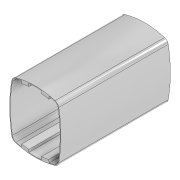
# Autodesk Inventor part: lineaire as deel 3
Saved by Autodesk Inventor 2020.3 (Build 243373000, 373)
## iProperties
Created: 2020-09-16
Part Number: lineaire as deel 3
Material: Aluminum 6061
Document SubType Name: Modeling
Designer: Svend
Density: 2.7 g/cm^3
Appearance: Aluminum - Polished
Author: Svend
Autodesk Inventor part; units mm, degrees
ref_plane "YZ Plane" through (0, 0, 0) normal (1, 0, 0) x (0, 1, 0)
ref_plane "XZ Plane" through (0, 0, 0) normal (0, 1, 0) x (-1, 0, 0)
ref_plane "XY Plane" through (0, 0, 0) normal (0, 0, 1) x (1, 0, 0)
sketch "Sketch1" plane through (0, 0, 0) normal (0, 0, 1) x (1, 0, 0)
  line L0 (-57, -57.5) -> (57, 57.5) construction
  line L1 (-67.5, 67.5) -> (67.5, 67.5) construction
  line L2 (67.5, 67.5) -> (67.5, -67.5) construction
  line L3 (67.5, -67.5) -> (-67.5, -67.5) construction
  line L4 (-67.5, -67.5) -> (-67.5, 67.5) construction
  line L5 (-67.5, 67.5) -> (67.5, -67.5) construction
  line L6 (67.5, 67.5) -> (-67.5, -67.5) construction
  circle A0 centre (-37.5, 37.5) radius 4
  circle A1 centre (-37.5, -37.5) radius 4
  circle A2 centre (37.5, -37.5) radius 4
  circle A3 centre (37.5, 37.5) radius 4
  arc A4 (-48.5, 62.5) -> (-48.5, -62.5) centre (326.325, 0) ccw
  line L7 (0, 67.5) -> (0, -67.5) construction
  line L8 (67.5, -67.5) -> (67.5, 67.5) construction
  arc A5 (48.5, -62.5) -> (48.5, 62.5) centre (-326.325, 0) ccw
  arc A6 (48.5, 62.5) -> (-48.5, 62.5) centre (0, -110.8429) ccw
  line L9 (-67.5, 0) -> (53.675, 0) construction
  arc A7 (-48.5, -62.5) -> (48.5, -62.5) centre (0, 110.8429) ccw
  arc A8 (-30.7003, 46.1842) -> (-30.7003, -46.1842) centre (326.325, 0) ccw
  arc A9 (-30.7003, -46.1842) -> (30.7003, -46.1842) centre (0, 110.8429) ccw
  arc A10 (30.7003, -46.1842) -> (30.7003, 46.1842) centre (-326.325, 0) ccw
  arc A11 (30.7003, 46.1842) -> (-30.7003, 46.1842) centre (0, -110.8429) ccw
  arc A12 (-55.5322, 68.7683) -> (-55.5322, -68.7683) centre (326.325, 0) ccw
  arc A13 (-55.5322, -68.7683) -> (55.5322, -68.7683) centre (0, 110.8429) ccw
  arc A14 (55.5322, -68.7683) -> (55.5322, 68.7683) centre (-326.325, 0) ccw
  arc A15 (55.5322, 68.7683) -> (-55.5322, 68.7683) centre (0, -110.8429) ccw
  arc A16 (-57.2838, 70.3161) -> (-57.2838, -70.3161) centre (326.325, 0) ccw
  arc A17 (-57.2838, -70.3161) -> (57.2838, -70.3161) centre (0, 110.8429) ccw
  arc A18 (57.2838, -70.3161) -> (57.2838, 70.3161) centre (-326.325, 0) ccw
  arc A19 (57.2838, 70.3161) -> (-57.2838, 70.3161) centre (0, -110.8429) ccw
  line L10 (18.657, 86.2762) -> (17.0881, 68.3442)
  line L11 (40.2153, 83.0301) -> (37.0881, 65.2948)
  line L12 (-18.657, 86.2762) -> (-17.0881, 68.3442)
  line L13 (-40.2153, 83.0301) -> (-37.0881, 65.2948)
  line L14 (18.657, -86.2762) -> (17.0881, -68.3442)
  line L15 (40.2153, -83.0301) -> (37.0881, -65.2948)
  line L16 (-40.2153, -83.0301) -> (-37.0881, -65.2948)
  line L17 (-18.657, -86.2762) -> (-17.0881, -68.3442)
  arc A20 (-64.266, 76.4373) -> (-64.266, -76.4373) centre (326.325, 0) ccw
  arc A21 (-64.266, -76.4373) -> (64.266, -76.4373) centre (0, 110.8429) ccw
  arc A22 (64.266, -76.4373) -> (64.266, 76.4373) centre (-326.325, 0) ccw
  arc A23 (64.266, 76.4373) -> (-64.266, 76.4373) centre (0, -110.8429) ccw
  arc A24 (-66.006, 77.9512) -> (-66.006, -77.9512) centre (326.325, 0) ccw
  arc A25 (-66.006, -77.9512) -> (66.006, -77.9512) centre (0, 110.8429) ccw
  arc A26 (66.006, -77.9512) -> (66.006, 77.9512) centre (-326.325, 0) ccw
  arc A27 (66.006, 77.9512) -> (-66.006, 77.9512) centre (0, -110.8429) ccw
  point P0 (0, 0)
  point P1 (0, 0)
  point P2 (-53.675, 0)
  point P3 (0, 0)
  point P4 (-17.7854, 76.314)
  point P5 (-38.478, 73.1774)
  point P6 (17.7854, -76.314)
  point P7 (38.478, -73.1774)
  point P8 (-38.478, -73.1774)
  point P9 (-17.7854, -76.314)
  point P10 (-38.478, 73.1774)
  point P11 (-17.7854, 76.314)
  point P12 (38.478, -73.1774)
  point P13 (17.7854, -76.314)
  point P14 (-17.7854, -76.314)
  point P15 (-38.478, -73.1774)
  point P16 (-17.9597, -78.3064)
  point P17 (-38.8255, -75.1479)
  point P18 (-38.8255, 75.1479)
  point P19 (-17.9597, 78.3064)
  point P20 (17.9597, 78.3064)
  point P21 (38.8255, 75.1479)
  point P22 (38.8255, -75.1479)
  point P23 (17.9597, -78.3064)
  dimension "d3" = 135
  dimension "d4" = 135
  dimension "d5" = 8
  dimension "d9" = 360
  dimension "d29" = 75
  dimension "d30" = 125
  dimension "d31" = 97
  dimension "d32" = 180
  dimension "d33" = 380
  dimension "d34" = 20
  dimension "d36" = 8
  dimension "d37" = 2
  dimension "d38" = 5
  dimension "d39" = 20
  dimension "d41" = 5
  dimension "d42" = 8
  dimension "d43" = 2
  constraints: 59 point on circle, 36 end point, 28 centre point, 13 symmetric about line, 7 midpoint, 7 point on line, 2 horizontal, 2 parallel, 1 coincident, 1 horizontal alignment, 1 perpendicular, 26 other
  measures "d3" distance of L2.end L3.end
  measures "d4" distance of L1.end L2.end
  measures "d5" diameter of A0
  measures "d29" distance of A0.centre A3.centre
  measures "d30" distance of A4.end A4.start
  measures "d31" distance of A5.end A4.start
  measures "d32" radius of A6
  measures "d33" radius of A4
  measures "d34" radial gap between concentric circles of A6 A11
  measures "d36" radial gap between concentric circles of A6 A15
  measures "d37" radial gap between concentric circles of A15 A19
  measures "d38" angle of L10 L11
  measures "d39" horizontal distance of L10.end L11.end
  measures "d41" angle of L7 L10
  measures "d42" radial gap between concentric circles of A19 A23
  measures "d43" radial gap between concentric circles of A23 A27
extrude "Extrusion1" add sketch "Sketch1" along normal mid plane 310 contours L13 A23 L12 A19 | A17 L17 A21 L16 | L10 A23 L11 A19 | A17 L15 A21 L14 | A27 A26 A25 A24
fillet "Fillet2" radius 15 8 edges at (64.266, 76.4373, 0) (-64.266, 76.4373, 0) (-64.266, -76.4373, 0) (64.266, -76.4373, 0) (-66.006, 77.9512, 0) (-66.006, -77.9512, 0) (66.006, -77.9512, 0) (66.006, 77.9512, 0)
sketch "Sketch4" plane through (0, 0, -155) normal (0, 0, -1) x (-1, 0, 0)
  arc A0 (67.6752, -69.0208) -> (67.6752, 69.0208) centre (-326.325, 0) ccw projected
  arc A1 (-57.1894, 80.8062) -> (-67.6752, 69.0208) centre (-52.9002, 66.4325) ccw projected
  arc A2 (-67.6752, 69.0208) -> (-67.6752, -69.0208) centre (326.325, 0) ccw projected
  arc A3 (-67.6752, -69.0208) -> (-57.1894, -80.8062) centre (-52.9002, -66.4325) ccw projected
  arc A4 (-57.1894, -80.8062) -> (57.1894, -80.8062) centre (0, 110.8429) ccw projected
  arc A5 (57.1894, -80.8062) -> (67.6752, -69.0208) centre (52.9002, -66.4325) ccw projected
  arc A6 (67.6752, -69.0208) -> (67.6752, 69.0208) centre (-326.325, 0) ccw projected
  arc A7 (67.6752, 69.0208) -> (57.1894, 80.8062) centre (52.9002, 66.4325) ccw projected
  arc A8 (57.1894, 80.8062) -> (-57.1894, 80.8062) centre (0, -110.8429) ccw projected
  line L0 (17.9597, -78.3064) -> (18.657, -86.2762) projected
  arc A9 (-18.657, -86.2762) -> (18.657, -86.2762) centre (0, 110.8429) ccw projected
  line L1 (-18.657, -86.2762) -> (-17.9597, -78.3064) projected
  arc A10 (-38.8255, -75.1479) -> (-17.9597, -78.3064) centre (0, 110.8429) ccw projected
  line L2 (-38.8255, -75.1479) -> (-40.2153, -83.0301) projected
  arc A11 (-55.3342, -79.268) -> (-40.2153, -83.0301) centre (0, 110.8429) ccw projected
  arc A12 (-65.9255, -67.4061) -> (-55.3342, -79.268) centre (-51.1422, -64.8656) ccw projected
  arc A13 (-65.9255, 67.4061) -> (-65.9255, -67.4061) centre (326.325, 0) ccw projected
  arc A14 (-55.3342, 79.268) -> (-65.9255, 67.4061) centre (-51.1422, 64.8656) ccw projected
  arc A15 (-40.2153, 83.0301) -> (-55.3342, 79.268) centre (0, -110.8429) ccw projected
  line L3 (-40.2153, 83.0301) -> (-38.8255, 75.1479) projected
  arc A16 (-17.9597, 78.3064) -> (-38.8255, 75.1479) centre (0, -110.8429) ccw projected
  line L4 (-17.9597, 78.3064) -> (-18.657, 86.2762) projected
  arc A17 (18.657, 86.2762) -> (-18.657, 86.2762) centre (0, -110.8429) ccw projected
  line L5 (18.657, 86.2762) -> (17.9597, 78.3064) projected
  arc A18 (38.8255, 75.1479) -> (17.9597, 78.3064) centre (0, -110.8429) ccw projected
  line L6 (38.8255, 75.1479) -> (40.2153, 83.0301) projected
  arc A19 (55.3342, 79.268) -> (40.2153, 83.0301) centre (0, -110.8429) ccw projected
  arc A20 (65.9255, 67.4061) -> (55.3342, 79.268) centre (51.1422, 64.8656) ccw projected
  arc A21 (65.9255, -67.4061) -> (65.9255, 67.4061) centre (-326.325, 0) ccw projected
  arc A22 (55.3342, -79.268) -> (65.9255, -67.4061) centre (51.1422, -64.8656) ccw projected
  arc A23 (40.2153, -83.0301) -> (55.3342, -79.268) centre (0, 110.8429) ccw projected
  line L7 (40.2153, -83.0301) -> (38.8255, -75.1479) projected
  arc A24 (17.9597, -78.3064) -> (38.8255, -75.1479) centre (0, 110.8429) ccw projected
  point P0 (0, 0)
  point P1 (67.6752, 69.0208)
extrude "Extrusion4" add sketch "Sketch4" along normal blind 5 contours A5 A4 A3 A2 A1 A8 A7 A0 | L0 A9 L1 A10 L2 A11 A12 A13 A14 A15 L3 A16 L4 A17 L5 A18 L6 A19 A20 A21 A22 A23 L7 A24
body "Solid1"
